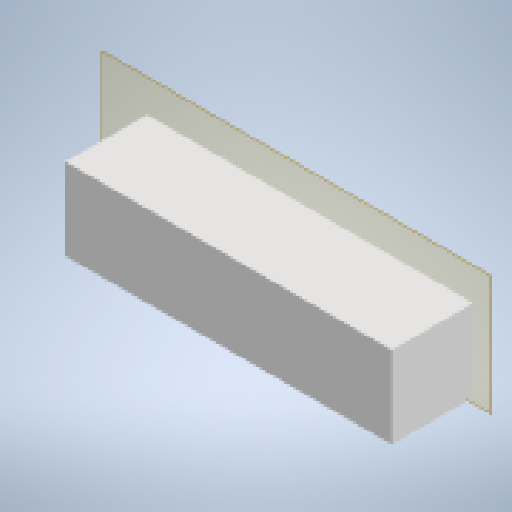
# Autodesk Inventor part: Coms
Saved by Autodesk Inventor 2027.1 (Build 311270010, 270A)
## iProperties
Created: 2026-09-10
Part Number: Coms
Material: Generic
Document SubType Name: Modeling
Designer: PWYNNE
Density: 1 g/cm^3
Appearance: Default
Author: PWYNNE
Autodesk Inventor part; units mm, degrees
ref_plane "YZ Plane" through (0, 0, 0) normal (1, 0, 0) x (0, 1, 0)
ref_plane "XZ Plane" through (0, 0, 0) normal (0, 1, 0) x (-1, 0, 0)
ref_plane "XY Plane" through (0, 0, 0) normal (0, 0, 1) x (1, 0, 0)
ref_plane "Work Plane1" through (0, 0, 0) normal (0, 0, 1) x (1, 0, 0)
sketch "Sketch1" plane through (0, 0, 0) normal (0, 0, 1) x (1, 0, 0)
  line L0 (10, -35) -> (10, 15) projected
  line L1 (0, 0) -> (130, 0) projected
  line L2 (130, 0) -> (130, 40) projected
  line L3 (0, 40) -> (130, 40) projected
  line L4 (0, 0) -> (0, 40) projected
  line L5 (130, 0) -> (10, 0)
  line L6 (10, 0) -> (10, 30)
  line L7 (10, 30) -> (130, 30)
  line L8 (130, 30) -> (130, 0)
  point P0 (10, 0)
  dimension "d0" = 30
  constraints: 8 end point, 2 parallel, 1 horizontal, 1 perpendicular
  measures "d0" distance of L5.end L6.end
extrude "Extrusion1" add sketch "Sketch1" along normal blind 30 contours L0 L6 L7 L2 L1
body "Solid1"
